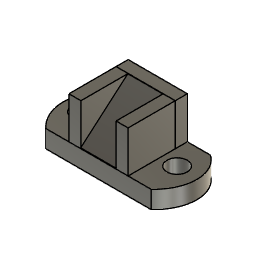
A2 (Autodesk Fusion 360 design; units mm, degrees)
Autodesk Fusion 360 part; units mm, degrees
sketch "Sketch1" plane through (0, 0, 0) normal (0, 0, 1) x (1, 0, 0)
  line L0 (0, 20) -> (-57, 20)
  line L1 (-57, 20) -> (-57, -44.0884)
  line L2 (-57, -44.0884) -> (0, -44.0884)
  line L3 (0, -44.0884) -> (0, 20)
  spline S0 degree 2 poles (-57, 20) (-95.6605, -7.4836) (-57, -44.0884) knots 0 0 0 7.117874 7.117874 7.117874 weights 1 0.666667 1
  line L4 (0, 14.9673) -> (0, 0)
  line L5 (57, 20) -> (57, -44.0884)
  line L6 (0, 20) -> (57, 20)
  line L7 (57, -44.0884) -> (0, -44.0884)
  line L8 (0, 14.9673) -> (0, 0)
  line L9 (0, -44.0884) -> (0, 20)
  spline S1 degree 2 poles (57, 20) (95.6605, -7.4836) (57, -44.0884) knots 0 0 0 7.117874 7.117874 7.117874 weights 1 0.666667 1
  dimension "d1" = 57
  constraint horizontal L0
  constraint vertical L1
  constraint horizontal L2
  constraint vertical L3
  constraint coincident L3 L4.start
  constraint coincident L4.end L8.end
  constraint vertical L4
  measures "d1" distance of L0.start L0.end
extrude "Extrude1" add sketch "Sketch1" along normal blind 19 makes body 1
hole "Hole1" at (49.231, -8.2942, 19) direction (0, 0, -1) diameter 22 depth 20 tip angle 118 bodies 1
hole "Hole2" at (-53.1008, -8.897, 19) direction (0, 0, -1) diameter 22 depth 20 tip angle 118 bodies 1
sketch "Sketch4" plane through (0, 0, 0) normal (0, 0, 1) x (1, 0, 0)
  line L0 (-32, 20) -> (32, 20)
  line L1 (32, 20) -> (32, 6.9575)
  line L2 (32, 6.9575) -> (-32, 6.9575)
  line L3 (-32, 6.9575) -> (-32, 20)
  dimension "d13" = 64
  constraint horizontal L0
  constraint vertical L1
  constraint horizontal L2
  constraint vertical L3
  measures "d13" distance of L0.start L0.end
extrude "Extrude2" add sketch "Sketch4" along normal blind 64 separate body makes body 2
sketch "Sketch5" plane through (0, 0, 0) normal (0, 0, 1) x (1, 0, 0)
  line L0 (-31.9975, 6.8685) -> (-18.9975, 6.8685)
  line L1 (-18.9975, 6.8685) -> (-18.9975, -44.0821)
  line L2 (-18.9975, -44.0821) -> (-31.9975, -44.0821)
  line L3 (-31.9975, -44.0821) -> (-31.9975, 6.8685)
  line L4 (31.9975, -44.0821) -> (31.9975, 6.8685)
  line L5 (31.9975, 6.8685) -> (18.9975, 6.8685)
  line L6 (18.9975, 6.8685) -> (18.9975, -44.0821)
  line L7 (18.9975, -44.0821) -> (31.9975, -44.0821)
  dimension "d16" = 13
  constraint horizontal L0
  constraint vertical L1
  constraint horizontal L2
  constraint vertical L3
  measures "d16" distance of L0.start L0.end
extrude "Extrude3" add sketch "Sketch5" along normal blind 64 separate body makes body 3 at (-18.9975, -10.1151, 21.3333) makes body 4 at (18.9975, -10.1151, 21.3333)
sketch "Sketch6" plane through (0, 0, 0) normal (1, 0, 0) x (0, 1, 0)
  line L0 (6.6698, 63.9302, -19) -> (6.6698, 20, -19)
  line L1 (-44.3302, 20, -19) -> (6.6698, 63.9302, -19)
  line L2 (-44.3302, 20, -19) -> (6.6698, 20, -19)
extrude "Extrude4" add sketch "Sketch6" along normal blind 38 separate body contours L0 L1 L2 in plane through (-19, 0, 0) normal (1, 0, 0) makes body 5
combine "Combine1" operation add target body 1 tool bodies 2 3 4 5 result as body 6 in component "Component"
delete_body "RemoveBody5" bodies 1
component "Component" placed x (1, 0, 0) y (0, 1, 0) z (0, 0, 1) at (0, 0, 0)
